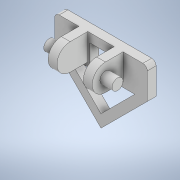
# Autodesk Inventor part: 02-2
Saved by Autodesk Inventor 2022 (Build 260153000, 153)
## iProperties
Created: 2021-09-12
Part Number: 02-2
Material: 일반
Document SubType Name: Modeling
Designer: 서울공업고등학교
Density: 1 g/cm^3
Appearance: 기본값
Author: 서울공업고등학교
Autodesk Inventor part; units mm, degrees
ref_plane "XZ Plane" through (0, 0, 0) normal (0, 1, 0) x (-1, 0, 0)
ref_plane "XY Plane" through (0, 0, 0) normal (0, 0, 1) x (1, 0, 0)
sketch "스케치1" plane through (0, 0, 0) normal (0, 0, 1) x (1, 0, 0)
  line L0 (0, 0) -> (0, 50)
  line L1 (0, 0) -> (50, 0) construction
  line L2 (0, 0) -> (-21, 21)
  line L3 (-21, 21) -> (-21, 35)
  line L4 (-21, 35) -> (0, 35)
  line L5 (0, 5.6569) -> (-15.3431, 21)
  line L6 (-15.3431, 21) -> (-5, 21)
  line L7 (-5, 21) -> (-5, 31)
  line L8 (-5, 31) -> (0, 31)
  line L9 (0, 0) -> (21, 21)
  line L10 (21, 21) -> (21, 35)
  line L11 (21, 35) -> (0, 35)
  line L12 (0, 5.6569) -> (15.3431, 21)
  line L13 (15.3431, 21) -> (5, 21)
  line L14 (5, 21) -> (5, 31)
  line L15 (5, 31) -> (0, 31)
  dimension "d0" = 50
  dimension "d2" = 35
  dimension "d3" = 45
  dimension "d4" = 4
  dimension "d5" = 10
  dimension "d6" = 42
  dimension "d7" = 10
  dimension "d8" = 4
  constraints: 32 end point, 5 symmetric about line, 4 perpendicular, 3 point on line, 2 parallel, 2 vertical, 1 horizontal
  measures "d0" distance of L0.start L0.end
  measures "d2" distance from line of L4 L0.start
  measures "d3" angle of L0 L2
  measures "d4" distance between parallel lines of L4 L8
  measures "d5" distance between parallel lines of L6 L8
  measures "d6" diameter of L3 L0
  measures "d7" diameter of L7 L0
  measures "d8" distance between parallel lines of L2 L5
extrude "돌출1" add sketch "스케치1" against normal blind 4 contours L2 L3 L4 L0 L8 L7 L6 L5 | L0 L12 L13 L14 L15 L11 L10 L9
ref_plane "작업 평면1" through (6, 0, 0) normal (1, 0, 0) x (0, 1, 0)
sketch "스케치2" plane through (6, 0, 0) normal (1, 0, 0) x (0, 1, 0)
  arc A0 (35, 8) -> (23, 8) centre (29, 8) ccw
  circle A1 centre (29, 8) radius 2.5
  line L0 (35, 0) -> (21, 0) projected
  line L1 (35, 0) -> (35, 8)
  line L2 (23, 8) -> (23, 0)
  line L3 (21, -4) -> (35, -4) projected
  point P0 (0, 0)
  dimension "d12" = 12
  dimension "d13" = 5
  dimension "d14" = 12
  dimension "d15" = 18
  dimension "d16" = 12
  constraints: 4 end point, 3 point on circle, 2 centre point, 2 point on line, 1 coincident, 1 parallel, 1 tangent, 1 vertical
  measures "d12" diameter of A0
  measures "d13" diameter of A1
  measures "d14" distance from line of L3 A0.centre
  measures "d16" distance between parallel lines of L2 L1
extrude "돌출2" add sketch "스케치2" along normal blind 4
extrude "돌출3" add sketch "스케치2" along normal blind 9.5 contours A1
mirror "미러1" about plane through (0, 0, 0) normal (1, 0, 0) of "돌출2", "돌출3"
fillet "모깎기1" radius 2 2 edges at (21, 35, -2) (-21, 35, -2)
